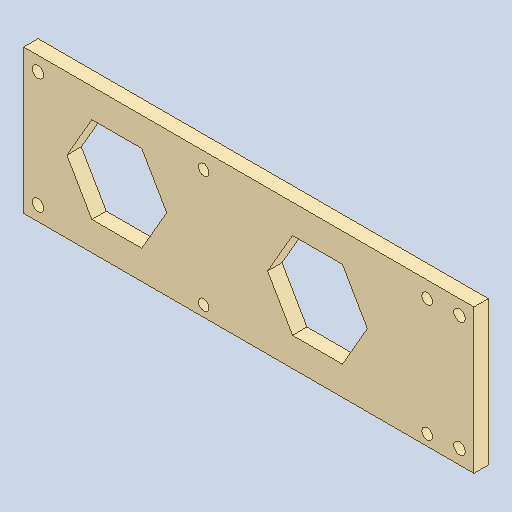
# Autodesk Inventor part: для_стаба
Saved by Autodesk Inventor 2023.1 (Build 271208000, 208)
## iProperties
Created: 2026-02-22
Part Number: для_стаба
Material: Типовые
Document SubType Name: Modeling
Designer: DELL
Density: 1 g/cm^3
Appearance: Бежевый
Author: DELL
Autodesk Inventor part; units mm, degrees
ref_plane "YZ Plane" through (0, 0, 0) normal (1, 0, 0) x (0, 1, 0)
ref_plane "XZ Plane" through (0, 0, 0) normal (0, 1, 0) x (-1, 0, 0)
ref_plane "XY Plane" through (0, 0, 0) normal (0, 0, 1) x (1, 0, 0)
sketch "Эскиз1" plane through (0, 0, 0) normal (0, 0, 1) x (1, 0, 0)
  line L0 (-62.5, 20) -> (62.5, 20)
  line L1 (62.5, 20) -> (62.5, -20)
  line L2 (62.5, -20) -> (-62.5, -20)
  line L3 (-62.5, -20) -> (-62.5, 20)
  line L4 (-62.5, 20) -> (62.5, -20) construction
  line L5 (62.5, 20) -> (-62.5, -20) construction
  point P0 (0, 0)
  dimension "d0" = 125
  dimension "d1" = 40
  constraints: 12 end point, 2 midpoint, 2 parallel, 1 horizontal, 1 perpendicular
  measures "d0" distance of L1.end L2.end
  measures "d1" distance of L0.end L1.end
extrude "Выдавливание1" add sketch "Эскиз1" along normal blind 4
sketch "Эскиз2" plane through (0, 0, 4) normal (0, 0, 1) x (1, 0, 0)
  circle A0 centre (-58.5, 16) radius 1.6
  line L0 (62.5, 20) -> (-62.5, 20) projected
  line L1 (-62.5, 20) -> (-62.5, -20) projected
  line L2 (-62.5, -20) -> (62.5, -20) construction
  line L3 (0, -20) -> (0, 0) construction
  line L4 (62.5, 0) -> (0, 0) construction
  circle A1 centre (58.5, 16) radius 1.6
  circle A2 centre (-58.5, -16) radius 1.6
  circle A3 centre (58.5, -16) radius 1.6
  dimension "d4" = 3.2
  dimension "d5" = 4
  dimension "d6" = 4
  constraints: 4 centre point, 4 end point, 3 symmetric about line, 1 midpoint, 1 perpendicular, 1 vertical, 3 other
  measures "d4" diameter of A0
  measures "d5" distance from line of L0 A0.centre
  measures "d6" distance from line of L1 A0.centre
extrude "Выдавливание2" cut sketch "Эскиз2" against normal blind 4
sketch "Эскиз3" plane through (0, 0, 0) normal (0, 0, -1) x (-1, 0, 0)
  circle A0 centre (-49.5, 15.5) radius 1.5 projected
  circle A1 centre (-49.5, -17) radius 1.5 projected
  circle A2 centre (12.5, 15.5) radius 1.5 projected
  circle A3 centre (12.5, -17) radius 1.5 projected
  line L0 (29.7154, -12) -> (22.7872, 0)
  line L1 (22.7872, 0) -> (29.7154, 12)
  line L2 (29.7154, 12) -> (43.5718, 12)
  line L3 (43.5718, 12) -> (50.5, 0)
  line L4 (50.5, 0) -> (43.5718, -12)
  line L5 (43.5718, -12) -> (29.7154, -12)
  line L6 (-62.5, 20) -> (62.5, 20) projected
  line L7 (62.5, -20) -> (-62.5, -20) projected
  line L8 (-5.2128, 0) -> (-12.141, -12)
  line L9 (-12.141, -12) -> (-25.9974, -12)
  line L10 (-25.9974, -12) -> (-32.9256, 0)
  line L11 (-32.9256, 0) -> (-25.9974, 12)
  line L12 (-25.9974, 12) -> (-12.141, 12)
  line L13 (-12.141, 12) -> (-5.2128, 0)
  line L14 (62.5, 20) -> (62.5, -20) projected
  point P0 (0, 0)
  point P1 (36.6436, 0)
  point P2 (-19.0692, 0)
  point P3 (-19.0692, -12)
  point P4 (62.5, 0)
  dimension "d10" = 8
  dimension "d11" = 8
  dimension "d12" = 8
  dimension "d13" = 8
  dimension "d14" = 28
  dimension "d15" = 12
  constraints: 24 end point, 2 midpoint, 1 parallel, 26 other
  measures "d10" distance between parallel lines of L6 L2
  measures "d11" distance between parallel lines of L7 L5
  measures "d12" distance between parallel lines of L6 L12
  measures "d13" distance from line of L7 point (-19.069, -12)
  measures "d14" distance of L0.end L8.start
  measures "d15" distance of point (62.5, 0) L3.end
extrude "Выдавливание3" cut sketch "Эскиз3" against normal blind 4
